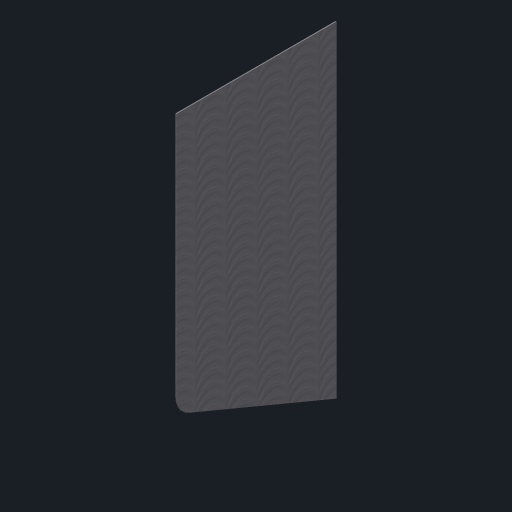
# Autodesk Inventor part: AUX_2
Saved by Autodesk Inventor 2024.3 (Build 283343000, 343)
## iProperties
Created: 2024-07-02
Part Number: AUX_2
Material: Steel, Mild, Welded
Document SubType Name: Modeling
Designer: Niler
Density: 7.85 g/cm^3
Appearance: Weld - Steel Mild
Author: Niler
Autodesk Inventor part; units mm, degrees
ref_plane "YZ Plane" through (0, 0, 0) normal (1, 0, 0) x (0, 1, 0)
ref_plane "XZ Plane" through (0, 0, 0) normal (0, 1, 0) x (-1, 0, 0)
ref_plane "XY Plane" through (0, 0, 0) normal (0, 0, 1) x (1, 0, 0)
sketch "Sketch1" plane through (0, 0, 0) normal (1, 0, 0) x (0, 1, 0)
  line L0 (648.272, -112.4756) -> (-626.3265, -112.4756)
  line L1 (648.272, -112.4756) -> (648.272, 120.9703)
  line L2 (-509.0568, 120.9703) -> (648.272, 120.9703)
  arc A0 (-509.0568, 120.9703) -> (-536.7491, 102.5088) centre (-509.0568, 90.9703) ccw
  line L3 (-626.3265, -112.4756) -> (-536.7491, 102.5088)
  line L4 (-150, 198.5295) -> (-150, -253.5175)
  point P0 (0, 0)
  point P1 (-150, 120.9703)
  point P2 (-150, -112.4756)
  dimension "d2" = 150
  constraints: 10 end point, 2 point on circle, 1 centre point, 1 perpendicular, 1 vertical
  measures "d2" distance from line of L4 point (0, 0)
extrude "Extrusion1" add sketch "Sketch1" along normal blind 1.5 contours L0 L3 A0 L2 L4
body "Solid1"
